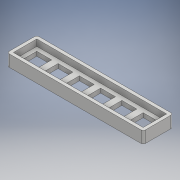
# Autodesk Inventor part: Key Plate Wide
Saved by Autodesk Inventor 2018 (Build 220112000, 112)
## iProperties
Created: 2018-05-10
Part Number: Key Plate Wide
Material: Generic
Document SubType Name: Modeling
Designer: mtsti
Density: 1 g/cm^3
Appearance: Default
Author: mtsti
Autodesk Inventor part; units mm, degrees
ref_plane "YZ Plane" through (0, 0, 0) normal (1, 0, 0) x (0, 1, 0)
ref_plane "XZ Plane" through (0, 0, 0) normal (0, 1, 0) x (-1, 0, 0)
ref_plane "XY Plane" through (0, 0, 0) normal (0, 0, 1) x (1, 0, 0)
sketch "Sketch7" plane through (0, 0, 0) normal (0, 0, 1) x (1, 0, 0)
  line L0 (-0.4948, 28.697) -> (127.5052, 28.697)
  line L1 (127.5052, 28.697) -> (127.5052, 56.697)
  line L2 (127.5052, 56.697) -> (-0.4948, 56.697)
  line L3 (-0.4948, 56.697) -> (-0.4948, 28.697)
  point P0 (0, 0)
  dimension "d136" = 128
  dimension "d137" = 28
  constraints: 8 end point, 2 parallel, 1 horizontal, 1 perpendicular
  measures "d136" distance of L2.end L1.end
  measures "d137" distance of L1.end L0.end
extrude "Extrusion6" add sketch "Sketch7" along normal blind 10
fillet "Fillet3" radius 2 4 edges at (-0.4948, 28.697, 5) (-0.4948, 56.697, 5) (127.5052, 28.697, 5) (127.5052, 56.697, 5)
sketch "Sketch8" plane through (0, 0, 10) normal (0, 0, 1) x (1, 0, 0)
  line L0 (2.5052, 31.697) -> (124.5052, 31.697)
  line L1 (124.5052, 31.697) -> (124.5052, 53.697)
  line L2 (124.5052, 53.697) -> (2.5052, 53.697)
  line L3 (2.5052, 53.697) -> (2.5052, 31.697)
  line L4 (125.5052, 56.697) -> (1.5052, 56.697) projected
  line L5 (-0.4948, 54.697) -> (-0.4948, 30.697) projected
  line L6 (1.5052, 28.697) -> (125.5052, 28.697) projected
  line L7 (127.5052, 30.697) -> (127.5052, 54.697) projected
  point P0 (0, 0)
  dimension "d141" = 3
  dimension "d142" = 3
  dimension "d143" = 3
  dimension "d144" = 3
  constraints: 8 end point, 2 parallel, 1 horizontal, 1 perpendicular
  measures "d141" distance between parallel lines of L4 L2
  measures "d142" distance between parallel lines of L5 L3
  measures "d143" distance between parallel lines of L6 L0
  measures "d144" distance between parallel lines of L7 L1
extrude "Extrusion7" cut sketch "Sketch8" against normal blind 6
sketch "Sketch9" plane through (0, 0, 4) normal (0, 0, 1) x (1, 0, 0)
  line L0 (6.5052, 35.697) -> (20.5052, 35.697)
  line L1 (20.5052, 35.697) -> (20.5052, 49.697)
  line L2 (20.5052, 49.697) -> (6.5052, 49.697)
  line L3 (6.5052, 49.697) -> (6.5052, 35.697)
  line L4 (26.5052, 35.697) -> (40.5052, 35.697)
  line L5 (40.5052, 35.697) -> (40.5052, 49.697)
  line L6 (40.5052, 49.697) -> (26.5052, 49.697)
  line L7 (26.5052, 49.697) -> (26.5052, 35.697)
  line L8 (46.5052, 35.697) -> (60.5052, 35.697)
  line L9 (60.5052, 35.697) -> (60.5052, 49.697)
  line L10 (60.5052, 49.697) -> (46.5052, 49.697)
  line L11 (46.5052, 49.697) -> (46.5052, 35.697)
  line L12 (66.5052, 35.697) -> (80.5052, 35.697)
  line L13 (80.5052, 35.697) -> (80.5052, 49.697)
  line L14 (80.5052, 49.697) -> (66.5052, 49.697)
  line L15 (66.5052, 49.697) -> (66.5052, 35.697)
  line L16 (86.5052, 35.697) -> (100.5052, 35.697)
  line L17 (100.5052, 35.697) -> (100.5052, 49.697)
  line L18 (100.5052, 49.697) -> (86.5052, 49.697)
  line L19 (86.5052, 49.697) -> (86.5052, 35.697)
  line L20 (106.5052, 35.697) -> (120.5052, 35.697)
  line L21 (120.5052, 35.697) -> (120.5052, 49.697)
  line L22 (120.5052, 49.697) -> (106.5052, 49.697)
  line L23 (106.5052, 49.697) -> (106.5052, 35.697)
  line L24 (2.5052, 31.697) -> (2.5052, 53.697) projected
  line L25 (124.5052, 53.697) -> (124.5052, 31.697) projected
  line L26 (2.5052, 53.697) -> (124.5052, 53.697) projected
  line L27 (124.5052, 31.697) -> (2.5052, 31.697) projected
  point P0 (0, 0)
  dimension "d147" = 14
  dimension "d148" = 14
  dimension "d149" = 14
  dimension "d150" = 14
  dimension "d151" = 14
  dimension "d152" = 14
  dimension "d153" = 14
  dimension "d154" = 14
  dimension "d155" = 14
  dimension "d156" = 14
  dimension "d157" = 14
  dimension "d158" = 14
  dimension "d159" = 4
  dimension "d160" = 6
  dimension "d161" = 6
  dimension "d162" = 6
  dimension "d163" = 6
  dimension "d164" = 6
  dimension "d165" = 4
  dimension "d166" = 4
  dimension "d167" = 4
  dimension "d168" = 4
  dimension "d169" = 4
  dimension "d170" = 4
  constraints: 48 end point, 13 equal length, 6 horizontal, 6 perpendicular, 2 point on line
  measures "d147" distance of L2.end L1.end
  measures "d148" distance of L1.end L0.end
  measures "d149" distance of L6.end L5.end
  measures "d150" distance of L5.end L4.end
  measures "d151" distance of L10.end L9.end
  measures "d152" distance of L9.end L8.end
  measures "d153" distance of L14.end L13.end
  measures "d154" distance of L13.end L12.end
  measures "d155" distance of L18.end L17.end
  measures "d156" distance of L17.end L16.end
  measures "d157" distance of L22.end L21.end
  measures "d158" distance of L21.end L20.end
  measures "d159" distance between parallel lines of L24 L3
  measures "d160" distance between parallel lines of L7 L1
  measures "d161" distance between parallel lines of L11 L5
  measures "d162" distance between parallel lines of L9 L15
  measures "d163" distance between parallel lines of L23 L17
  measures "d164" distance between parallel lines of L13 L19
  measures "d165" distance between parallel lines of L25 L21
  measures "d166" distance between parallel lines of L26 L2
  measures "d167" distance between parallel lines of L27 L0
  measures "d168" distance between parallel lines of L6 L26
  measures "d169" distance between parallel lines of L26 L14
  measures "d170" distance between parallel lines of L26 L22
extrude "Extrusion8" cut sketch "Sketch9" against normal blind 4 contours L3 L2 L1 L0 | L7 L6 L5 L4 | L11 L10 L9 L8 | L15 L14 L13 L12 | L19 L18 L17 L16 | L23 L22 L21 L20
sketch "Sketch11" plane through (0, 0, 0) normal (0, 0, -1) x (-1, 0, 0)
  line L0 (0.4948, 28.697) -> (-127.5052, 28.697)
  line L1 (-127.5052, 28.697) -> (-127.5052, 56.697)
  line L2 (-127.5052, 56.697) -> (0.4948, 56.697)
  line L3 (0.4948, 56.697) -> (0.4948, 28.697)
  line L4 (-127.5052, 30.697) -> (-127.5052, 54.697) projected
  line L5 (-125.5052, 56.697) -> (-1.5052, 56.697) projected
  line L6 (-1.5052, 28.697) -> (-125.5052, 28.697) projected
  line L7 (0.4948, 54.697) -> (0.4948, 30.697) projected
  line L8 (-126.0052, 30.197) -> (-1.0052, 30.197)
  line L9 (-1.0052, 30.197) -> (-1.0052, 55.197)
  line L10 (-1.0052, 55.197) -> (-126.0052, 55.197)
  line L11 (-126.0052, 55.197) -> (-126.0052, 30.197)
  point P0 (0, 0)
  dimension "d173" = 0
  dimension "d174" = 0
  dimension "d175" = 0
  dimension "d176" = 0
  dimension "d177" = 1.5
  dimension "d178" = 1.5
  dimension "d179" = 1.5
  dimension "d180" = 1.5
  constraints: 16 end point, 4 parallel, 2 horizontal, 2 perpendicular
  measures "d173" distance between parallel lines of L4 L1
  measures "d174" distance between parallel lines of L5 L2
  measures "d175" distance between parallel lines of L6 L0
  measures "d176" distance between parallel lines of L7 L3
  measures "d177" distance between parallel lines of L4 L11
  measures "d178" distance between parallel lines of L0 L8
  measures "d179" distance between parallel lines of L2 L10
  measures "d180" distance between parallel lines of L3 L9
extrude "Extrusion9" add sketch "Sketch11" along normal blind 1
fillet "Fillet4" radius 2 4 edges at (-0.4948, 28.697, -0.5) (127.5052, 56.697, -0.5) (127.5052, 28.697, -0.5) (-0.4948, 56.697, -0.5)
body "Solid2"
